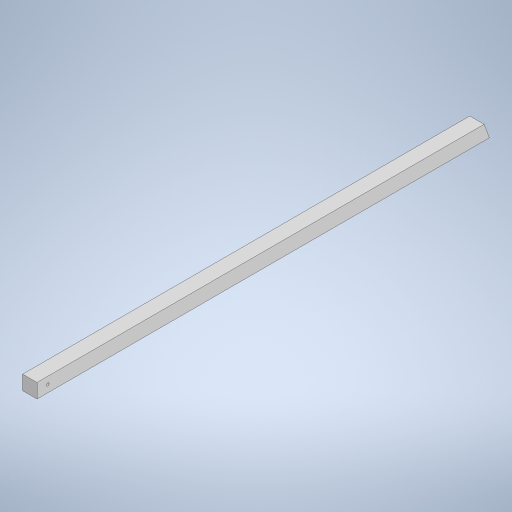
# Autodesk Inventor part: VersaFrame 1x1 ( support corssbars )
Saved by Autodesk Inventor 2023 (Build 270158000, 158)
## iProperties
Created: 2023-01-23
Part Number: VersaFrame 1x1 ( support corssbars )
Material: Generic
Document SubType Name: Modeling
Designer: Gabriel - T3 CAD
Density: 1 g/cm^3
Appearance: Default
Author: Gabriel - T3 CAD
Autodesk Inventor part; units mm, degrees
ref_plane "YZ Plane" through (0, 0, 0) normal (1, 0, 0) x (0, 1, 0)
ref_plane "XZ Plane" through (0, 0, 0) normal (0, 1, 0) x (-1, 0, 0)
ref_plane "XY Plane" through (0, 0, 0) normal (0, 0, 1) x (1, 0, 0)
sketch "Sketch1" plane through (0, 0, 0) normal (0, 0, 1) x (1, 0, 0)
  line L0 (0, 0) -> (-25.4, 0)
  line L1 (-25.4, 0) -> (-25.4, 25.4)
  line L2 (-25.4, 25.4) -> (0, 25.4)
  line L3 (0, 25.4) -> (0, 0)
  dimension "d0" = 25.4
  dimension "d1" = 25.4
  constraints: 8 end point, 2 parallel, 1 horizontal, 1 perpendicular
  measures "d0" distance of L1.end L2.end
  measures "d1" distance of L0.end L1.end
extrude "Extrusion1" add sketch "Sketch1" along normal blind 800.1
sketch "Sketch2" plane through (0, 0, 0) normal (1, 0, 0) x (0, 0, -1)
  circle A0 centre (-781.05, 12.7) radius 2.3813
  line L0 (0, 25.4) -> (-800.1, 25.4) projected
  line L1 (-800.1, 0) -> (-800.1, 25.4) projected
  line L2 (0, 0) -> (-800.1, 0) projected
  line L3 (0, 0) -> (0, 25.4) projected
  line L4 (0, 0) -> (-9.2448, 25.4)
  line L5 (0, 25.4) -> (-800.1, 25.4) projected
  line L6 (0, 0) -> (27.0301, 0) construction
  point P0 (-800.1, 12.7)
  dimension "d4" = 12.7
  dimension "d5" = 19.05
  dimension "d6" = 4.7625
  dimension "d12" = 110
  constraints: 4 end point, 1 centre point, 1 equal length, 1 horizontal, 1 midpoint, 1 point on line
  measures "d4" distance from line of A0.centre L0
  measures "d5" distance of point (-800.1, 12.7) A0.centre
  measures "d6" diameter of A0
  measures "d12" angle of L6 L4
extrude "Extrusion2" cut sketch "Sketch2" against normal through all contours A0 | L3 L4 L0
body "Solid1"
